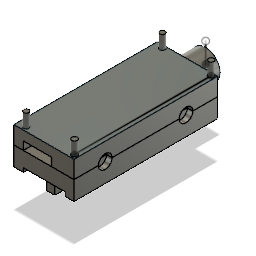
Atari 7800 mod Stand v7 (Autodesk Fusion 360 design; units mm, degrees)
Autodesk Fusion 360 part; units mm, degrees
sketch "Sketch1" plane through (0, 0, 0) normal (0, 1, 0) x (1, 0, 0)
  circle A0 centre (10, -10) radius 1
  circle A1 centre (26.65, -10) radius 1
  circle A2 centre (26.65, -58.45) radius 1
  circle A3 centre (10, -58.45) radius 1
  dimension "d1" = 2
  dimension "d3" = 16.65
  dimension "d4" = 2
  dimension "d5" = 48.45
  dimension "d6" = 2
  dimension "d7" = 2
  measures "d1" diameter of A0
  measures "d3" distance of A0.centre A1.centre
  measures "d4" diameter of A1
  measures "d5" distance of A1.centre A2.centre
  measures "d6" diameter of A2
  measures "d7" diameter of A3
extrude "Extrude1" add sketch "Sketch1" along normal blind 5 makes body 1 at (27.6488, 3.3333, 10.0498) makes body 2 at (9.0603, 3.3333, 58.792) makes body 3 at (10.9988, 3.3333, 10.0498) makes body 4 at (27.5897, 3.3333, 58.792)
sketch "Sketch3" plane through (0, 0, 0) normal (0, 1, 0) x (1, 0, 0)
  line L0 (9, -9) -> (28, -9)
  line L1 (28, -9) -> (28, -60)
  line L2 (28, -60) -> (9, -60)
  line L3 (9, -60) -> (9, -9)
  constraint horizontal L0
  constraint vertical L1
  constraint horizontal L2
  constraint vertical L3
extrude "Extrude2" add sketch "Sketch3" against normal blind 1 bodies 1 2 3 4
sketch "Sketch6" plane through (0, 0, 9) normal (0, 0, -1) x (-1, 0, 0)
  line L0 (-9, 0) -> (-10, 0)
  line L1 (-10, 0) -> (-26.65, 0)
  line L2 (-26.65, 0) -> (-28, 0)
  line L3 (-28, 0) -> (-28, -1)
  line L4 (-28, -1) -> (-9, -1)
  line L5 (-9, -1) -> (-9, 0)
  line L6 (-25.65, 0) -> (-14.65, 0)
  line L7 (-14.65, 0) -> (-14.65, -2)
  circle A0 centre (-14.65, -7.3) radius 5.3
  point P0 (-25.65, 0)
  dimension "d12" = 11
  dimension "d13" = 2
  dimension "d14" = 10.6
  constraint coincident P0 L6.start
  constraint coincident L7.end A0
  measures "d12" distance of P0 L6.end
  measures "d13" distance of L6.end L7.end
  measures "d14" diameter of A0
extrude "Extrude3" add sketch "Sketch6" against normal blind 24.4 separate body contours A0 makes body 5
sketch "Sketch7" plane through (0, 0, 33.4) normal (0, 0, 1) x (1, 0, 0)
  circle A0 centre (14.65, -7.3) radius 5.3
  circle A1 centre (14.65, -7.3) radius 4.625
  circle A2 centre (14.65, -7.3) radius 3.85
  line L0 (14.65, -7.3) -> (19.275, -7.3)
  line L1 (14.65, -7.3) -> (10.025, -7.3)
  line L2 (10.025, -7.3) -> (14.65, -7.3)
  line L3 (14.65, -7.3) -> (14.65, -2.675)
  line L4 (14.65, -7.3) -> (14.65, -11.925)
  line L5 (14.65, -3.45) -> (12.0872, -3.45)
  line L6 (12.0872, -3.45) -> (14.65, -3.45)
  line L7 (17.2128, -3.45) -> (14.65, -3.45)
  line L8 (14.65, -11.15) -> (17.2128, -11.15)
  line L9 (14.65, -11.15) -> (12.0872, -11.15)
  constraint concentric A0 A1
  constraint concentric A1 A2
  constraint coincident A0.centre A1.centre
  constraint coincident A1 L0.end
  constraint coincident A1 L1.end
  constraint parallel L0 L1
  constraint coincident A1 L3.end
  constraint perpendicular L0 L3
  constraint coincident A1 L4.end
  constraint perpendicular L2 L4
  constraint coincident A2 L5.start
  constraint coincident L3 L5.start
  constraint coincident A1 L5.end
  constraint tangent A2 L5
  constraint coincident A1 L7.start
  constraint tangent A2 L7
  constraint coincident A2 L8.start
  constraint coincident L4 L8.start
  constraint coincident A1 L8.end
  constraint tangent A2 L8
  constraint coincident A1 L9.end
  constraint tangent A2 L9
extrude "Extrude4" add sketch "Sketch7" along normal blind 13 contours A1 A2 L0 L7 | A1 A2 L0 L8 | A2 L0 L3 | A2 L0 L4 | A2 L1 L2 L3 | A1 A2 L1 L2 L5 L6 | A1 A2 L1 L2 L9 | A2 L1 L2 L4 bodies 5
sketch "Sketch8" plane through (0, -11.15, 0) normal (0, -1, 0) x (1, 0, 0)
  line L0 (12.0872, 33.4) -> (17.2128, 33.4)
  line L1 (17.2128, 33.4) -> (17.2128, 46.4)
  line L2 (17.2128, 46.4) -> (12.0872, 46.4)
  line L3 (12.0872, 46.4) -> (12.0872, 33.4)
  line L4 (14.65, 46.4) -> (14.65, 44.4)
  line L5 (14.65, 33.4) -> (14.65, 37.4)
  line L6 (14.65, 37.4) -> (19.65, 37.4)
  line L7 (19.65, 37.4) -> (19.65, 38.7)
  line L8 (19.65, 38.7) -> (14.65, 38.7)
  line L9 (14.65, 38.7) -> (14.65, 37.4)
  line L10 (14.65, 44.4) -> (19.65, 44.4)
  line L11 (19.65, 44.4) -> (19.65, 43.1)
  line L12 (19.65, 43.1) -> (14.65, 43.1)
  line L13 (14.65, 43.1) -> (14.65, 44.4)
  line L14 (14.65, 41.5) -> (19.65, 41.5)
  line L15 (19.65, 41.5) -> (19.65, 40.2)
  line L16 (19.65, 40.2) -> (14.65, 40.2)
  line L17 (14.65, 40.2) -> (14.65, 41.5)
  line L18 (14.65, 44.4) -> (9.65, 44.4)
  line L19 (9.65, 44.4) -> (9.65, 43.1)
  line L20 (9.65, 43.1) -> (14.65, 43.1)
  line L21 (14.65, 43.1) -> (14.65, 44.4)
  line L22 (14.65, 41.5) -> (9.65, 41.5)
  line L23 (9.65, 41.5) -> (9.65, 40.2)
  line L24 (9.65, 40.2) -> (14.65, 40.2)
  line L25 (14.65, 40.2) -> (14.65, 41.5)
  line L26 (14.65, 38.7) -> (9.65, 38.7)
  line L27 (9.65, 38.7) -> (9.65, 37.4)
  line L28 (9.65, 37.4) -> (14.65, 37.4)
  line L29 (14.65, 37.4) -> (14.65, 38.7)
  dimension "d21" = 2
  dimension "d26" = 4
  dimension "d27" = 5
  dimension "d28" = 1.3
  dimension "d29" = 5
  dimension "d30" = 1.3
  dimension "d31" = 1.6
  dimension "d32" = 5
  dimension "d33" = 1.3
  dimension "d34" = 5
  dimension "d35" = 5
  dimension "d36" = 1.3
  dimension "d37" = 1.3
  dimension "d38" = 5
  constraint midpoint L2 L4.start
  constraint midpoint L0 L5.start
  constraint horizontal L6
  constraint vertical L7
  constraint horizontal L8
  constraint vertical L9
  constraint horizontal L10
  constraint vertical L11
  constraint horizontal L12
  constraint vertical L13
  constraint horizontal L14
  constraint vertical L15
  constraint horizontal L16
  constraint vertical L17
  constraint horizontal L18
  constraint vertical L19
  constraint horizontal L20
  constraint vertical L21
  constraint horizontal L22
  constraint vertical L23
  constraint horizontal L24
  constraint vertical L25
  constraint horizontal L26
  constraint vertical L27
  constraint horizontal L28
  constraint vertical L29
  measures "d21" distance of L4.start L4.end
  measures "d26" distance of L5.start L5.end
  measures "d27" distance of L5.end L6.end
  measures "d28" distance of L5.end L8.end
  measures "d29" distance of L4.end L10.end
  measures "d30" distance of L4.end L12.end
  measures "d31" distance of L12.end L14.start
  measures "d32" distance of L14.start L14.end
  measures "d33" distance of L14.start L16.end
  measures "d34" distance of L4.end L18.end
  measures "d35" distance of L14.start L22.end
  measures "d36" distance of L14.start L16.end
  measures "d37" distance of L8.end L5.end
  measures "d38" distance of L8.end L26.end
extrude "Extrude5" cut sketch "Sketch8" against normal blind 3 contours L3 L26 L27 L28 | L3 L9 L26 L28 L29 | L1 L6 L8 L9 L29 | L1 L6 L7 L8 | L3 L22 L23 L24 | L3 L17 L22 L24 L25 | L1 L14 L16 L17 L25 | L1 L14 L15 L16 | L3 L18 L19 L20 | L3 L13 L18 L20 L21 | L1 L10 L12 L13 L21 | L1 L10 L11 L12 bodies 5
sketch "Sketch9" plane through (0, -3.45, 0) normal (0, 1, 0) x (-1, 0, 0)
  line L0 (-17.2128, 33.4) -> (-12.0872, 33.4)
  line L1 (-12.0872, 33.4) -> (-12.0872, 46.4)
  line L2 (-12.0872, 46.4) -> (-17.2128, 46.4)
  line L3 (-17.2128, 46.4) -> (-17.2128, 33.4)
  line L4 (-19.1962, 44.4) -> (-10.1038, 44.4)
  line L5 (-10.1038, 44.4) -> (-10.1038, 43.1)
  line L6 (-10.1038, 43.1) -> (-19.1962, 43.1)
  line L7 (-19.1962, 43.1) -> (-19.1962, 44.4)
  line L8 (-10.1038, 41.5) -> (-19.1962, 41.5)
  line L9 (-19.1962, 41.5) -> (-19.1962, 40.2)
  line L10 (-19.1962, 40.2) -> (-10.1038, 40.2)
  line L11 (-10.1038, 40.2) -> (-10.1038, 41.5)
  line L12 (-19.1962, 38.7) -> (-10.1038, 38.7)
  line L13 (-10.1038, 38.7) -> (-10.1038, 37.4)
  line L14 (-10.1038, 37.4) -> (-19.1962, 37.4)
  line L15 (-19.1962, 37.4) -> (-19.1962, 38.7)
  point P0 (-19.1962, 44.4)
  point P1 (-10.1038, 43.1)
  point P2 (-10.1038, 41.5)
  point P3 (-19.1962, 40.2)
  point P4 (-19.1962, 38.7)
  point P5 (-10.1038, 37.4)
  constraint horizontal L4
  constraint vertical L5
  constraint horizontal L6
  constraint vertical L7
  constraint coincident P1 L5.end
  constraint coincident P0 L4.start
  constraint horizontal L8
  constraint vertical L9
  constraint horizontal L10
  constraint vertical L11
  constraint coincident P3 L9.end
  constraint coincident P2 L8.start
  constraint horizontal L12
  constraint vertical L13
  constraint horizontal L14
  constraint vertical L15
  constraint coincident P5 L13.end
  constraint coincident P4 L12.start
extrude "Extrude6" cut sketch "Sketch9" against normal blind 3 contours L3 L12 L14 L15 | L1 L3 L12 L14 | L1 L12 L13 L14 | L3 L8 L9 L10 | L1 L3 L8 L10 | L1 L8 L10 L11 | L3 L4 L6 L7 | L1 L3 L4 L6 | L1 L4 L5 L6 bodies 5
move_body "Move2" bodies 5 to x (1, 0, 0) y (0, 1, 0) z (0, 0, 1) at (0, 0, -9)
sketch "Sketch10" plane through (0, 5, 0) normal (0, 1, 0) x (-1, 0, 0)
  circle A0 centre (-26.65, 10) radius 1
sketch "Sketch11" plane through (0, 0, 0) normal (0, 0, 1) x (1, 0, 0)
  line L0 (5, 5) -> (5, -23.5)
  line L1 (5, -23.5) -> (35, -23.5)
  line L2 (35, -23.5) -> (35, -25)
  line L3 (35, -25) -> (5, -25)
  line L4 (5, -25) -> (5, -23.5)
  dimension "d43" = 28.5
  dimension "d44" = 30
  constraint horizontal L1
  constraint vertical L2
  constraint horizontal L3
  constraint vertical L4
  measures "d43" distance of L0.start L0.end
  measures "d44" distance of L0.end L1.end
extrude "Extrude7" add sketch "Sketch11" along normal blind 66 separate body makes body 6
extrude "Extrude8" add 1 faces at (15.3333, -1, 26) along direction (0, -1, 0) blind 1 on bodies 1 bodies 1
sketch "Sketch12" plane through (0, 0, 60) normal (0, 0, 1) x (1, 0, 0)
  line L0 (28, 0) -> (9, 0)
  line L1 (9, 0) -> (9, -2)
  line L2 (9, -2) -> (28, -2)
  line L3 (28, -2) -> (28, 0)
  line L4 (9, -2) -> (17.2128, -2)
  line L5 (17.2128, -2) -> (17.2128, -3.45)
  line L6 (17.2128, -3.45) -> (9, -3.45)
  line L7 (9, -3.45) -> (9, -2)
  line L8 (17.2128, -3.45) -> (28, -3.45)
  line L9 (28, -3.45) -> (28, -2)
  line L10 (28, -2) -> (17.2128, -2)
  line L11 (17.2128, -2) -> (17.2128, -3.45)
  point P0 (17.2128, -3.45)
  point P1 (17.2128, -3.45)
  constraint horizontal L4
  constraint vertical L5
  constraint horizontal L6
  constraint vertical L7
  constraint coincident P1 P0
  constraint coincident L1.end L2.start
  constraint horizontal L8
  constraint vertical L9
  constraint horizontal L10
  constraint vertical L11
  constraint coincident L2.end L3.start
extrude "Extrude9" add sketch "Sketch12" against normal blind 35 contours L2 L5 L8 L9 L10 L11 | L2 L4 L5 L6 L7 L11 bodies 1
sketch "Sketch13" plane through (0, -3.45, 0) normal (0, -1, 0) x (1, 0, 0)
  line L0 (28, 60) -> (9, 60)
  line L1 (9, 60) -> (9, 25)
  line L2 (9, 25) -> (28, 25)
  line L3 (28, 25) -> (28, 60)
  line L4 (9, 25) -> (10, 25)
  line L5 (10, 25) -> (10, 60)
  line L6 (10, 60) -> (9, 60)
  line L7 (9, 60) -> (9, 25)
  line L8 (28, 25) -> (19.3, 25)
  line L9 (19.3, 25) -> (19.3, 35.4)
  line L10 (19.3, 35.4) -> (28, 35.4)
  line L11 (28, 35.4) -> (28, 25)
  line L12 (19.3, 35.4) -> (28, 35.4)
  line L13 (28, 35.4) -> (28, 60)
  line L14 (28, 60) -> (19.3, 60)
  line L15 (19.3, 60) -> (19.3, 35.4)
  constraint horizontal L4
  constraint vertical L5
  constraint horizontal L6
  constraint vertical L7
  constraint coincident L0 L5.end
  constraint coincident L1.end L2.start
  constraint horizontal L8
  constraint vertical L9
  constraint horizontal L10
  constraint vertical L11
  constraint coincident L2.end L3.start
  constraint horizontal L12
  constraint vertical L13
  constraint horizontal L14
  constraint vertical L15
  constraint coincident L0.start L3.end
extrude "Extrude10" add sketch "Sketch13" along normal blind 4 contours L0 L3 L10 L12 L13 L14 L15 | L2 L3 L8 L9 L10 L11 L12 | L0 L1 L2 L4 L5 L6 L7 bodies 1
sketch "Sketch14" plane through (0, 0, 9) normal (0, 0, -1) x (-1, 0, 0)
  line L0 (-9, 0) -> (-10, 0)
  line L1 (-10, 0) -> (-26.65, 0)
  line L2 (-26.65, 0) -> (-28, 0)
  line L3 (-28, 0) -> (-28, -2)
  line L4 (-28, -2) -> (-9, -2)
  line L5 (-9, -2) -> (-9, 0)
  line L6 (-9, -2) -> (-28, -2)
  line L7 (-28, -2) -> (-28, -7.45)
  line L8 (-28, -7.45) -> (-9, -7.45)
  line L9 (-9, -7.45) -> (-9, -2)
  circle A0 centre (-14.65, -7.2999) radius 5.3001
  circle A1 centre (-14.65, -7.3) radius 5.3
  point P0 (-28, -7.45)
  constraint horizontal L6
  constraint vertical L7
  constraint horizontal L8
  constraint vertical L9
  constraint coincident P0 L7.end
  constraint coincident L4.end L5.start
  constraint tangent A0 A1
extrude "Extrude11" add sketch "Sketch14" against normal blind 16 contours L4 L6 L8 L9 A0 A1 | L4 L6 L7 L8 A0 A1 bodies 1
sketch "Sketch15" plane through (0, -3.45, 0) normal (0, -1, 0) x (1, 0, 0)
  line L0 (10, 60) -> (10, 25)
  line L1 (10, 25) -> (11.0072, 25)
  line L2 (11.0072, 25) -> (18.2928, 25)
  line L3 (18.2928, 25) -> (19.3, 25)
  line L4 (19.3, 25) -> (19.3, 60)
  line L5 (19.3, 60) -> (10, 60)
  line L6 (10.1038, 35.4) -> (19.1962, 35.4)
  line L7 (19.1962, 35.4) -> (19.1962, 34.1)
  line L8 (19.1962, 34.1) -> (10.1038, 34.1)
  line L9 (10.1038, 34.1) -> (10.1038, 35.4)
  line L10 (19.1962, 32.5) -> (10.1038, 32.5)
  line L11 (10.1038, 32.5) -> (10.1038, 31.2)
  line L12 (10.1038, 31.2) -> (19.1962, 31.2)
  line L13 (19.1962, 31.2) -> (19.1962, 32.5)
  line L14 (10.1038, 29.7) -> (19.1962, 29.7)
  line L15 (19.1962, 29.7) -> (19.1962, 28.4)
  line L16 (19.1962, 28.4) -> (10.1038, 28.4)
  line L17 (10.1038, 28.4) -> (10.1038, 29.7)
  point P0 (10.1038, 35.4)
  point P1 (19.1962, 34.1)
  point P2 (19.1962, 32.5)
  point P3 (10.1038, 31.2)
  point P4 (10.1038, 29.7)
  point P5 (19.1962, 28.4)
  constraint horizontal L6
  constraint vertical L7
  constraint horizontal L8
  constraint vertical L9
  constraint coincident P1 L7.end
  constraint coincident P0 L6.start
  constraint horizontal L10
  constraint vertical L11
  constraint horizontal L12
  constraint vertical L13
  constraint coincident P3 L11.end
  constraint coincident P2 L10.start
  constraint horizontal L14
  constraint vertical L15
  constraint horizontal L16
  constraint vertical L17
  constraint coincident P5 L15.end
  constraint coincident P4 L14.start
extrude "Extrude12" add sketch "Sketch15" along normal blind 3 contours L6 L7 L8 L9 | L10 L11 L12 L13 | L14 L15 L16 L17 bodies 1
extrude "Extrude13" cut 4 faces at (9.4507, -7.45, 48.3333) (9.1174, -7.45, 14.3333) (22.416, -7.45, 48.3333) (25.316, -7.45, 14.3333) along direction (0, 1, 0) blind 1 on bodies 1 bodies 1
sketch "Sketch16" plane through (0, 0, 9) normal (0, 0, -1) x (-1, 0, 0)
  line L0 (-9.352, -6.45) -> (-9, -6.45)
  line L1 (-9, -6.45) -> (-9, 0)
  line L2 (-9, 0) -> (-10, 0)
  line L3 (-10, 0) -> (-26.65, 0)
  line L4 (-26.65, 0) -> (-28, 0)
  line L5 (-28, 0) -> (-28, -6.45)
  line L6 (-28, -6.45) -> (-19.948, -6.45)
  line L7 (-19.948, -6.45) -> (-19.948, -7.1498)
  arc A0 (-14.7005, -2) -> (-19.948, -7.1498) centre (-14.65, -7.2999) ccw
  line L8 (-14.7005, -2) -> (-14.5995, -2)
  arc A1 (-9.352, -7.1498) -> (-14.5995, -2) centre (-14.65, -7.2999) ccw
  line L9 (-9.352, -7.1498) -> (-9.352, -6.45)
  line L10 (-9, -6.45) -> (-21.6476, -6.45)
  line L11 (-21.6476, -6.45) -> (-21.6476, -7.1824)
  line L12 (-21.6476, -7.1824) -> (-9, -7.1824)
  line L13 (-9, -7.1824) -> (-9, -6.45)
  constraint horizontal L10
  constraint vertical L11
  constraint horizontal L12
  constraint vertical L13
  constraint coincident L0.end L1.start
extrude "Extrude14" cut 1 faces at (9.3521, -6.9152, 19.6667) along direction (1, 0, 0) blind 1 on bodies 1 bodies 1
extrude "Extrude15" cut 1 faces at (19.9479, -6.9151, 19.6667) along direction (-1, 0, 0) blind 1 on bodies 1 bodies 1
sketch "Sketch17" plane through (0, -6.45, 0) normal (0, -1, 0) x (1, 0, 0)
  line L0 (28, 9) -> (28, 60)
  line L1 (28, 60) -> (19.3, 60)
  line L2 (19.3, 60) -> (19.3, 25)
  line L3 (19.3, 25) -> (19.8815, 25)
  line L4 (19.8815, 25) -> (19.8815, 9)
  line L5 (19.8815, 9) -> (28, 9)
  line L6 (28, 9) -> (19.3, 9)
  line L7 (19.3, 9) -> (19.3, 60)
  line L8 (19.3, 60) -> (28, 60)
  line L9 (28, 60) -> (28, 9)
  line L10 (9, 9) -> (10, 9)
  line L11 (10, 9) -> (10, 60)
  line L12 (10, 60) -> (9, 60)
  line L13 (9, 60) -> (9, 9)
  point P0 (9, 9)
  point P1 (10, 60)
  constraint horizontal L6
  constraint vertical L7
  constraint horizontal L8
  constraint vertical L9
  constraint coincident L1.end L2.start
  constraint coincident L0.start L5.end
  constraint horizontal L10
  constraint vertical L11
  constraint horizontal L12
  constraint vertical L13
  constraint coincident P1 L11.end
  constraint coincident P0 L10.start
extrude "Extrude16" add sketch "Sketch17" along normal blind 2 separate body contours L0 L1 L2 L3 L4 L5 L6 L7 L8 L9 | L10 L11 L12 L13 makes body 7 at (25.2938, -6.45, 31.3333) makes body 8 at (9, -7.1167, 43)
sketch "Sketch18" plane through (0, -8.45, 0) normal (0, -1, 0) x (1, 0, 0)
  line L0 (19.3, 25) -> (19.8815, 25)
  line L1 (19.8815, 25) -> (19.8815, 9)
  line L2 (19.8815, 9) -> (28, 9)
  line L3 (28, 9) -> (28, 60)
  line L4 (28, 60) -> (19.3, 60)
  line L5 (19.3, 60) -> (19.3, 25)
  line L6 (19.1962, 35.4) -> (19.1962, 34.1)
  line L7 (19.1962, 34.75) -> (28, 34.7618)
  line L8 (28, 34.7618) -> (28, 35.2618)
  line L9 (28, 35.2618) -> (9, 35.2618)
  line L10 (9, 35.2618) -> (9, 34.2618)
  line L11 (9, 34.2618) -> (28, 34.2618)
  line L12 (28, 34.2618) -> (28, 35.2618)
  line L13 (19.1962, 32.5) -> (10.1038, 32.5)
  line L14 (10.1038, 32.5) -> (10.1038, 31.2)
  line L15 (10.1038, 31.2) -> (19.1962, 31.2)
  line L16 (10.1038, 29.7) -> (19.1962, 29.7)
  line L17 (19.1962, 28.4) -> (10.1038, 28.4)
  line L18 (10.1038, 28.4) -> (10.1038, 29.7)
  line L19 (19.1962, 31.85) -> (28, 31.8539)
  line L20 (19.1962, 29.05) -> (28, 29)
  line L21 (28, 29) -> (28, 29.5)
  line L22 (28, 31.8539) -> (28, 32.3539)
  line L23 (28, 29.5) -> (9, 29.5)
  line L24 (9, 29.5) -> (9, 28.5)
  line L25 (9, 28.5) -> (28, 28.5)
  line L26 (28, 28.5) -> (28, 29.5)
  line L27 (28, 32.3539) -> (9, 32.3539)
  line L28 (9, 32.3539) -> (9, 31.3539)
  line L29 (9, 31.3539) -> (28, 31.3539)
  line L30 (28, 31.3539) -> (28, 32.3539)
  line L31 (9, 60) -> (10, 60)
  line L32 (10, 60) -> (10, 9)
  line L33 (10, 9) -> (9, 9)
  line L34 (9, 9) -> (9, 60)
  point P0 (19.1962, 32.5)
  point P1 (10.1038, 31.2)
  point P2 (10.1038, 29.7)
  point P3 (19.1962, 28.4)
  point P4 (9, 60)
  point P5 (10, 9)
  dimension "d65" = 0.5
  dimension "d66" = 1
  dimension "d67" = 0.5
  dimension "d68" = 0.5
  dimension "d69" = 1
  dimension "d70" = 1
  constraint midpoint L6 L7.start
  constraint coincident L3 L7.end
  constraint horizontal L9
  constraint vertical L10
  constraint horizontal L11
  constraint vertical L12
  constraint horizontal L13
  constraint vertical L14
  constraint horizontal L15
  constraint coincident P1 L14.end
  constraint coincident P0 L13.start
  constraint horizontal L16
  constraint horizontal L17
  constraint vertical L18
  constraint coincident P3 L17.start
  constraint coincident P2 L16.start
  constraint coincident L3 L19.end
  constraint coincident L3 L20.end
  constraint horizontal L23
  constraint vertical L24
  constraint horizontal L25
  constraint vertical L26
  constraint horizontal L27
  constraint vertical L28
  constraint horizontal L29
  constraint vertical L30
  constraint horizontal L31
  constraint vertical L32
  constraint horizontal L33
  constraint vertical L34
  constraint coincident P5 L32.end
  constraint coincident P4 L31.start
  measures "d65" distance of L7.end L8.end
  measures "d66" distance of L8.end L11.end
  measures "d67" distance of L20.end L21.end
  measures "d68" distance of L19.end L22.end
  measures "d69" distance of L21.end L25.end
  measures "d70" distance of L22.end L29.end
extrude "Extrude17" add sketch "Sketch18" along normal blind 3 contours L0 L1 L2 L3 L5 L25 | L5 L18 L23 L25 | L3 L5 L20 L25 L26 | L3 L5 L20 L21 L23 L26 | L3 L5 L23 L29 | L25 L32 L33 L34 | L23 L24 L25 L32 L34 | L5 L14 L27 L29 | L3 L5 L19 L29 L30 | L23 L29 L32 L34 | L3 L5 L19 L22 L27 L30 | L27 L28 L29 L32 L34 | L3 L5 L11 L27 | L11 L27 L32 L34 | L3 L5 L7 L11 L12 | L6 L9 L11 L32 | L9 L10 L11 L32 L34 | L3 L5 L7 L8 L9 L12 | L9 L31 L32 L34 | L3 L4 L5 L9 bodies 8 makes body 9 at (25.1, -8.45, 33.7846)
extrude "Extrude18" add 1 faces at (10.1038, -9.45, 32.0206) along direction (-1, 0, 0) blind 1 on bodies 9 bodies 9 8
extrude "Extrude19" add 1 faces at (10.1038, -9.45, 28.8333) along direction (-1, 0, 0) blind 0.3 on bodies 9 bodies 9
extrude "Extrude20" add 1 faces at (19.1962, -9.45, 34.9285) along direction (1, 0, 0) blind 0.3 on bodies 9 bodies 9
extrude "Extrude21" add 1 faces at (25.2938, -8.45, 31.3333) along direction (0, -1, 0) blind 1 on bodies 7 bodies 7 9
sketch "Sketch19" plane through (19.3, 0, 0) normal (-1, 0, 0) x (0, 0, 1)
  line L0 (60, -11.45) -> (60, -6.45)
  line L1 (60, -6.45) -> (25, -6.45)
  line L2 (25, -6.45) -> (25, -11.45)
  line L3 (25, -11.45) -> (28.5, -11.45)
  line L4 (28.5, -11.45) -> (28.5, -8.45)
  line L5 (28.5, -8.45) -> (29.5, -8.45)
  line L6 (29.5, -8.45) -> (29.5, -11.45)
  line L7 (29.5, -11.45) -> (31.3539, -11.45)
  line L8 (31.3539, -11.45) -> (31.3539, -8.45)
  line L9 (31.3539, -8.45) -> (32.3539, -8.45)
  line L10 (32.3539, -8.45) -> (32.3539, -11.45)
  line L11 (32.3539, -11.45) -> (34.2618, -11.45)
  line L12 (34.2618, -11.45) -> (34.2618, -8.45)
  line L13 (34.2618, -8.45) -> (35.2618, -8.45)
  line L14 (35.2618, -8.45) -> (35.2618, -11.45)
  line L15 (35.2618, -11.45) -> (60, -11.45)
  line L16 (60, -11.45) -> (58, -11.45)
  line L17 (58, -11.45) -> (58, -6.45)
  line L18 (58, -6.45) -> (60, -6.45)
  line L19 (60, -6.45) -> (60, -11.45)
  dimension "d81" = 2
  constraint horizontal L16
  constraint vertical L17
  constraint horizontal L18
  constraint vertical L19
  constraint coincident L0.start L15.end
  measures "d81" distance of L0.start L16.end
extrude "Extrude22" add sketch "Sketch19" along normal blind 10 contours L0 L1 L15 L16 L17 L18 L19 bodies 7
sketch "Sketch20" plane through (28, 0, 0) normal (1, 0, 0) x (0, 0, -1)
  line L0 (-60, -6.45) -> (-9, -6.45)
  line L1 (-9, -6.45) -> (-9, 0)
  line L2 (-9, 0) -> (-60, 0)
  line L3 (-60, 0) -> (-60, -6.45)
  circle A0 centre (-50.0734, -6.45) radius 2.5
  circle A1 centre (-20.5371, -6.45) radius 2.5
  dimension "d84" = 5
  dimension "d85" = 5
  constraint coincident L0 A0.centre
  constraint coincident L0 A1.centre
  measures "d84" diameter of A0
  measures "d85" diameter of A1
extrude "Extrude23" cut sketch "Sketch20" against normal blind 2 contours L0 A1 | L0 A1 | L0 A0 | L0 A0 bodies 1 7
sketch "Sketch21" plane through (9, 0, 0) normal (-1, 0, 0) x (0, 0, 1)
  line L0 (60, -6.45) -> (9, -6.45)
  line L1 (9, -6.45) -> (9, -11.45)
  line L2 (9, -11.45) -> (60, -11.45)
  line L3 (60, -11.45) -> (60, -6.45)
  circle A0 centre (52.5734, -6.45) radius 2.5
  circle A1 centre (18.0371, -6.45) radius 2.5
  point P0 (52.5734, -6.45)
  point P1 (18.0371, -6.45)
  dimension "d88" = 5
  dimension "d89" = 5
  constraint coincident P0 A0.centre
  constraint coincident P1 A1.centre
  measures "d88" diameter of A0
  measures "d89" diameter of A1
extrude "Extrude24" cut sketch "Sketch21" against normal blind 0.7 contours L0 A0 | L0 A0 bodies 1 7
extrude "Extrude25" add 1 faces at (25.2938, -11.45, 31.3333) along direction (0, -1, 0) blind 2 on bodies 7 bodies 7
sketch "Sketch22" plane through (0, -13.45, 0) normal (0, -1, 0) x (1, 0, 0)
  line L0 (28, 60) -> (9, 60)
  line L1 (9, 60) -> (9, 9)
  line L2 (9, 9) -> (10, 9)
  line L3 (10, 9) -> (10, 28.5)
  line L4 (10, 28.5) -> (19.3, 28.5)
  line L5 (19.3, 28.5) -> (19.3, 25)
  line L6 (19.3, 25) -> (19.8815, 25)
  line L7 (19.8815, 25) -> (19.8815, 9)
  line L8 (19.8815, 9) -> (28, 9)
  line L9 (28, 9) -> (28, 60)
  line L10 (10, 29.5) -> (10, 31.3539)
  line L11 (10, 31.3539) -> (19.3, 31.3539)
  line L12 (19.3, 31.3539) -> (19.3, 29.5)
  line L13 (19.3, 29.5) -> (10, 29.5)
  line L14 (10, 34.2618) -> (19.3, 34.2618)
  line L15 (19.3, 34.2618) -> (19.3, 32.3539)
  line L16 (19.3, 32.3539) -> (10, 32.3539)
  line L17 (10, 32.3539) -> (10, 34.2618)
  line L18 (10, 58) -> (19.3, 58)
  line L19 (19.3, 58) -> (19.3, 35.2618)
  line L20 (19.3, 35.2618) -> (10, 35.2618)
  line L21 (10, 35.2618) -> (10, 58)
  line L22 (10, 60) -> (23.7, 60)
  line L23 (23.7, 60) -> (23.7, 34.3)
  line L24 (23.7, 34.3) -> (10, 34.3)
  line L25 (10, 34.3) -> (10, 60)
  point P0 (10, 60)
  dimension "d94" = 13.7
  dimension "d95" = 25.7
  constraint horizontal L22
  constraint vertical L23
  constraint horizontal L24
  constraint vertical L25
  constraint coincident P0 L22.start
  measures "d94" distance of P0 L22.end
  measures "d95" distance of P0 L24.end
extrude "Extrude26" cut sketch "Sketch22" against normal blind 1.5 contours L0 L18 L19 L20 L22 L23 L24 L25 | L18 L19 L20 L21 L25 bodies 7
sketch "Sketch23" plane through (0, -13.45, 0) normal (0, -1, 0) x (1, 0, 0)
  line L0 (10, 34.3) -> (10, 60)
  line L1 (10, 60) -> (9, 60)
  line L2 (9, 60) -> (9, 9)
  line L3 (9, 9) -> (10, 9)
  line L4 (10, 9) -> (10, 28.5)
  line L5 (10, 28.5) -> (19.3, 28.5)
  line L6 (19.3, 28.5) -> (19.3, 25)
  line L7 (19.3, 25) -> (19.8815, 25)
  line L8 (19.8815, 25) -> (19.8815, 9)
  line L9 (19.8815, 9) -> (28, 9)
  line L10 (28, 9) -> (28, 60)
  line L11 (28, 60) -> (23.7, 60)
  line L12 (23.7, 60) -> (23.7, 34.3)
  line L13 (23.7, 34.3) -> (10, 34.3)
  line L14 (10, 29.5) -> (10, 31.3539)
  line L15 (10, 31.3539) -> (19.3, 31.3539)
  line L16 (19.3, 31.3539) -> (19.3, 29.5)
  line L17 (19.3, 29.5) -> (10, 29.5)
  line L18 (10, 34.2618) -> (19.3, 34.2618)
  line L19 (19.3, 34.2618) -> (19.3, 32.3539)
  line L20 (19.3, 32.3539) -> (10, 32.3539)
  line L21 (10, 32.3539) -> (10, 34.2618)
  line L22 (19.3, 34.2618) -> (10, 34.2618)
  line L23 (10, 34.2618) -> (10, 28.5)
  line L24 (10, 28.5) -> (19.3, 28.5)
  line L25 (19.3, 28.5) -> (19.3, 34.2618)
  line L26 (19.3, 34.2618) -> (10, 34.2618)
  line L27 (10, 34.2618) -> (10, 34.3)
  line L28 (10, 34.3) -> (19.3, 34.3)
  line L29 (19.3, 34.3) -> (19.3, 34.2618)
  constraint horizontal L22
  constraint vertical L23
  constraint horizontal L24
  constraint vertical L25
  constraint coincident L4.end L5.start
  constraint coincident L18.end L19.start
  constraint horizontal L26
  constraint vertical L27
  constraint horizontal L28
  constraint vertical L29
  constraint coincident L0.start L13.end
extrude "Extrude27" cut sketch "Sketch23" against normal blind 1.5 contours L13 L18 L22 L26 L27 L28 L29 | L18 L19 L20 L21 L22 L23 L25 L26 | L15 L20 L23 L25 | L14 L15 L16 L17 L23 L25 | L5 L17 L23 L24 L25 bodies 7
sketch "Sketch24" plane through (0, 0, 9) normal (0, 0, -1) x (-1, 0, 0)
  line L0 (-19.8815, -13.45) -> (-19.8815, -6.45)
  line L1 (-19.8815, -6.45) -> (-28, -6.45)
  line L2 (-28, -6.45) -> (-28, -13.45)
  line L3 (-28, -13.45) -> (-19.8815, -13.45)
  line L4 (-28, -6.45) -> (-9, -6.45)
  line L5 (-9, -6.45) -> (-9, -13.45)
  line L6 (-9, -13.45) -> (-28, -13.45)
  line L7 (-28, -13.45) -> (-28, -6.45)
  circle A0 centre (-14.6632, -7.2997) radius 5.3001
  circle A1 centre (-14.65, -7.3) radius 5.3
  point P0 (-9, -13.45)
  point P1 (-14.5995, -2)
  constraint horizontal L4
  constraint vertical L5
  constraint horizontal L6
  constraint vertical L7
  constraint coincident P0 L5.end
  constraint coincident L1.end L2.start
  constraint coincident A0 P1
extrude "Extrude28" add sketch "Sketch24" against normal blind 16 contours L0 L1 L2 L3 L4 L6 L7 A0 | L0 L4 L5 L6 A0 A1 bodies 7
extrude "Extrude29" cut sketch "Sketch20" against normal blind 2 contours L0 A1 picked at (-20.5624, -7.5266) bodies 7
extrude "Extrude30" add 2 faces at (9, -4.8425, 33.3671) (9, -4.9667, 14.3333) along direction (-1, 0, 0) blind 1 on bodies 1 bodies 1
extrude "Extrude31" add 1 faces at (9, -8.9075, 22.7004) along direction (-1, 0, 0) blind 1 on bodies 7 bodies 7
move_face "MoveFace1" to x (1, 0, 0) y (0, 1, 0) z (0, 0, 1) at (-0.9876, 0, 0.1568) 2 faces at (10, 3.3333, 9) (9.6815, 5, 9.9017) on bodies 1
move_face "MoveFace2" to x (1, 0, 0) y (0, 1, 0) z (0, 0, 1) at (-1, 0, 0) 2 faces at (10.2554, 5, 58.8247) (10.995, 1.6667, 58.3504) on bodies 1
extrude "Extrude32" add 1 faces at (25.1, -3.3, 60) along direction (0, 0, 1) blind 1.5 on bodies 1 bodies 1
move_face "MoveFace3" to x (1, 0, 0) y (0, 1, 0) z (0, 0, 1) at (0, 0, 1.5) 2 faces at (9.2554, 5, 58.8247) (8.0012, 3.3333, 58.4002) on bodies 1
move_face "MoveFace4" to x (1, 0, 0) y (0, 1, 0) z (0, 0, 1) at (0, 0, 1.5) 2 faces at (26.9867, 5, 58.5946) (27.6488, 1.6667, 58.4002) on bodies 1
extrude "Extrude33" add 1 faces at (19.9, -8.2833, 60) along direction (0, 0, 1) blind 1.5 on bodies 7 bodies 7
extrude "Extrude34" cut 1 faces at (23.7, -12.95, 43.3667) along direction (1, 0, 0) blind 1 on bodies 7 bodies 7
sketch "Sketch25" plane through (0, 0, 0) normal (0, 0, -1) x (-1, 0, 0)
  circle A0 centre (-14.65, -7.3) radius 5.3
  circle A1 centre (-14.65, -7.3) radius 5.5
  dimension "d114" = 11
  constraint concentric A0 A1
  measures "d114" diameter of A1
extrude "Extrude35" cut sketch "Sketch25" against normal blind 25 contours A0 | A1 bodies 1 7
extrude "Extrude36" cut 1 faces at (16.1654, -4.45, 28.4) along direction (0, 0, 1) blind 0.15 on bodies 1 bodies 1
extrude "Extrude37" cut 1 faces at (13.1346, -4.45, 31.2) along direction (0, 0, 1) blind 0.15 on bodies 1 bodies 1
extrude "Extrude38" cut 1 faces at (16.1654, -4.45, 34.1) along direction (0, 0, 1) blind 0.15 on bodies 1 bodies 1
extrude "Extrude39" cut 1 faces at (13.1346, -4.45, 29.7) along direction (0, 0, -1) blind 0.15 on bodies 1 bodies 1
extrude "Extrude40" cut 1 faces at (16.1654, -4.45, 32.5) along direction (0, 0, -1) blind 0.15 on bodies 1 bodies 1
extrude "Extrude41" cut 1 faces at (13.1346, -4.45, 35.4) along direction (0, 0, -1) blind 0.15 on bodies 1 bodies 1
extrude "Extrude42" add 3 faces at (10.1038, -4.45, 34.5833) (10.1038, -4.45, 32.0167) (10.1038, -4.45, 28.8833) along direction (-1, 0, 0) blind 1 on bodies 1 bodies 1
extrude "Extrude43" add 3 faces at (19.1962, -4.45, 34.9167) (19.1962, -4.45, 31.6833) (19.1962, -4.45, 29.2167) along direction (1, 0, 0) blind 1 on bodies 1 bodies 1
extrude "Extrude44" cut 4 faces at (10, -4.8855, 27.3667) (10, -4.45, 30.15) (10, -5.45, 33.6167) (10, -4.45, 52.75) along direction (-1, 0, 0) blind 0.5 on bodies 1 bodies 1
extrude "Extrude45" cut 4 faces at (19.3, -4.8855, 27.3667) (19.3, -4.45, 30.15) (19.3, -5.45, 33.6167) (19.3, -4.45, 52.75) along direction (1, 0, 0) blind 0.5 on bodies 1 bodies 1
extrude "Extrude46" cut 1 faces at (19.3, -8.95, 50.4206) along direction (1, 0, 0) blind 0.5 on bodies 7 bodies 7
extrude "Extrude47" cut 1 faces at (10, -8.95, 50.4206) along direction (-1, 0, 0) blind 0.5 on bodies 7 bodies 7
sketch "Sketch26" plane through (9.5, 0, 0) normal (1, 0, 0) x (0, 0, -1)
  line L0 (-28.5, -11.95) -> (-29.5, -11.95)
  line L1 (-29.5, -11.95) -> (-29.5, -8.45)
  line L2 (-29.5, -8.45) -> (-28.5, -8.45)
  line L3 (-28.5, -8.45) -> (-28.5, -11.95)
  line L4 (-31.3539, -11.95) -> (-32.3539, -11.95)
  line L5 (-32.3539, -11.95) -> (-32.3539, -8.45)
  line L6 (-32.3539, -8.45) -> (-31.3539, -8.45)
  line L7 (-31.3539, -8.45) -> (-31.3539, -11.95)
  line L8 (-34.2618, -11.95) -> (-35.2618, -11.95)
  line L9 (-35.2618, -11.95) -> (-35.2618, -8.45)
  line L10 (-35.2618, -8.45) -> (-34.2618, -8.45)
  line L11 (-34.2618, -8.45) -> (-34.2618, -11.95)
  arc A0 (-55.0734, -6.45) -> (-50.0734, -6.45) centre (-52.5734, -6.45) ccw
  line L12 (-55.0734, -6.45) -> (-58, -6.45)
  line L13 (-58, -6.45) -> (-58, -11.95)
  line L14 (-58, -11.95) -> (-61.5, -11.95)
  line L15 (-61.5, -11.95) -> (-61.5, -13.45)
  line L16 (-61.5, -13.45) -> (-25, -13.45)
  line L17 (-25, -13.45) -> (-25, -9.2307)
  line L18 (-25, -9.2307) -> (-25, -6.45)
  line L19 (-25, -6.45) -> (-50.0734, -6.45)
  line L20 (-55.0734, -6.45) -> (-49.0947, -6.45)
  line L21 (-49.0947, -6.45) -> (-49.0947, -9.1965)
  line L22 (-49.0947, -9.1965) -> (-55.0734, -9.1965)
  line L23 (-55.0734, -9.1965) -> (-55.0734, -6.45)
  constraint horizontal L20
  constraint vertical L21
  constraint horizontal L22
  constraint vertical L23
  constraint coincident A0.start L12.start
extrude "Extrude48" add sketch "Sketch26" against normal blind 0.5 contours A0 L20 bodies 7
sketch "Sketch27" plane through (9.5, 0, 0) normal (1, 0, 0) x (0, 0, -1)
  arc A0 (-50.0734, -6.45) -> (-55.0734, -6.45) centre (-52.5734, -6.45) ccw
  line L0 (-50.0734, -6.45) -> (-35.25, -6.45)
  line L1 (-35.25, -6.45) -> (-35.25, -3.45)
  line L2 (-35.25, -3.45) -> (-61.5, -3.45)
  line L3 (-61.5, -3.45) -> (-61.5, -6.45)
  line L4 (-61.5, -6.45) -> (-55.0734, -6.45)
  line L5 (-55.0734, -6.45) -> (-49.9978, -6.45)
  line L6 (-49.9978, -6.45) -> (-49.9978, -3.45)
  line L7 (-49.9978, -3.45) -> (-55.0734, -3.45)
  line L8 (-55.0734, -3.45) -> (-55.0734, -6.45)
  constraint horizontal L5
  constraint vertical L6
  constraint horizontal L7
  constraint vertical L8
  constraint coincident L2 L6.end
  constraint coincident A0.end L4.end
extrude "Extrude49" add sketch "Sketch27" against normal blind 0.5 contours A0 L5 bodies 1
extrude "Extrude50" add 1 faces at (8, -4.1758, 22.7004) along direction (-1, 0, 0) blind 2 on bodies 1 bodies 1
extrude "Extrude51" add 1 faces at (8, -8.9075, 22.7004) along direction (-1, 0, 0) blind 2 on bodies 7 bodies 7
sketch "Sketch28" plane through (6, 0, 0) normal (-1, 0, 0) x (0, 0, 1)
  line L0 (9, -13.45) -> (61.5, -13.45)
  line L1 (61.5, -13.45) -> (61.5, -6.45)
  line L2 (61.5, -6.45) -> (55.0734, -6.45)
  arc A0 (50.0734, -6.45) -> (55.0734, -6.45) centre (52.5734, -6.45) ccw
  line L3 (50.0734, -6.45) -> (9, -6.45)
  line L4 (9, -6.45) -> (9, -13.45)
  line L5 (9, -13.45) -> (22.5, -13.45)
  line L6 (22.5, -13.45) -> (22.5, -26.95)
  line L7 (22.5, -26.95) -> (9, -26.95)
  line L8 (9, -26.95) -> (9, -13.45)
  line L9 (9, -20.2) -> (22.5, -20.2)
  line L10 (22.5, -13.45) -> (36, -13.45)
  line L11 (36, -13.45) -> (36, -26.95)
  line L12 (36, -26.95) -> (22.5, -26.95)
  line L13 (22.5, -26.95) -> (22.5, -13.45)
  line L14 (29.25, -13.45) -> (29.25, -26.95)
  line L15 (36, -13.45) -> (49.5, -13.45)
  line L16 (49.5, -13.45) -> (49.5, -26.95)
  line L17 (49.5, -26.95) -> (36, -26.95)
  line L18 (36, -26.95) -> (36, -13.45)
  line L19 (36, -20.2) -> (49.5, -20.2)
  circle A1 centre (15.75, -20.2) radius 3.1
  circle A2 centre (29.25, -20.2) radius 3.1
  circle A3 centre (42.75, -20.2) radius 3.1
  dimension "d149" = 13.5
  dimension "d150" = 13.5
  dimension "d151" = 13.5
  dimension "d152" = 13.5
  dimension "d153" = 13.5
  dimension "d154" = 13.5
  dimension "d155" = 6.2
  dimension "d156" = 6.2
  dimension "d157" = 6.2
  constraint horizontal L5
  constraint vertical L6
  constraint horizontal L7
  constraint vertical L8
  constraint coincident L0.start L4.end
  constraint midpoint L8 L9.start
  constraint midpoint L6 L9.end
  constraint horizontal L10
  constraint vertical L11
  constraint horizontal L12
  constraint vertical L13
  constraint midpoint L10 L14.start
  constraint midpoint L12 L14.end
  constraint horizontal L15
  constraint vertical L16
  constraint horizontal L17
  constraint vertical L18
  constraint midpoint L11 L19.start
  constraint midpoint L16 L19.end
  constraint midpoint L9 A1.centre
  constraint midpoint L14 A2.centre
  constraint midpoint L19 A3.centre
  measures "d149" distance of L0.start L5.end
  measures "d150" distance of L0.start L7.end
  measures "d151" distance of L5.end L10.end
  measures "d152" distance of L5.end L6.end
  measures "d153" distance of L10.end L15.end
  measures "d154" distance of L10.end L11.end
  measures "d155" diameter of A1
  measures "d156" diameter of A2
  measures "d157" diameter of A3
extrude "Extrude52" add sketch "Sketch28" against normal blind 3 contours L0 L5 L6 L8 L9 L13 A1 | L0 L6 L10 L12 L13 L14 A2 | L6 L7 L8 L9 L13 A1 | L0 L10 L11 L12 L14 L18 A2 | L0 L11 L15 L16 L18 L19 A3 | L11 L16 L17 L18 L19 A3 bodies 7
sketch "Sketch29" plane through (0, -6.45, 0) normal (0, -1, 0) x (1, 0, 0)
  line L0 (9.5, 34.25) -> (19.8, 34.25)
  line L1 (19.8, 34.25) -> (19.8, 32.35)
  line L2 (19.8, 32.35) -> (9.5, 32.35)
  line L3 (9.5, 32.35) -> (9.5, 34.25)
  line L4 (9.5, 31.35) -> (19.8, 31.35)
  line L5 (19.8, 31.35) -> (19.8, 29.55)
  line L6 (19.8, 29.55) -> (9.5, 29.55)
  line L7 (9.5, 29.55) -> (9.5, 31.35)
  line L8 (9.5, 35.25) -> (9.5, 61.5)
  line L9 (9.5, 61.5) -> (6, 61.5)
  line L10 (6, 61.5) -> (6, 55.0734)
  line L11 (6, 55.0734) -> (9, 55.0734)
  line L12 (9, 55.0734) -> (9, 50.0734)
  line L13 (9, 50.0734) -> (6, 50.0734)
  line L14 (6, 50.0734) -> (6, 9)
  line L15 (6, 9) -> (9.2161, 9)
  line L16 (9.2161, 9) -> (9.2161, 25)
  line L17 (9.2161, 25) -> (9.5, 25)
  line L18 (9.5, 25) -> (9.5, 28.55)
  line L19 (9.5, 28.55) -> (19.8, 28.55)
  line L20 (19.8, 28.55) -> (19.8, 25)
  line L21 (19.8, 25) -> (20.0839, 25)
  line L22 (20.0839, 25) -> (20.0839, 9)
  line L23 (20.0839, 9) -> (28, 9)
  line L24 (28, 9) -> (28, 18.0371)
  line L25 (28, 18.0371) -> (26, 18.0371)
  line L26 (26, 18.0371) -> (26, 23.0371)
  line L27 (26, 23.0371) -> (28, 23.0371)
  line L28 (28, 23.0371) -> (28, 47.5734)
  line L29 (28, 47.5734) -> (26, 47.5734)
  line L30 (26, 47.5734) -> (26, 52.5734)
  line L31 (26, 52.5734) -> (28, 52.5734)
  line L32 (28, 52.5734) -> (28, 61.5)
  line L33 (28, 61.5) -> (19.8, 61.5)
  line L34 (19.8, 61.5) -> (19.8, 35.25)
  line L35 (19.8, 35.25) -> (9.5, 35.25)
  line L36 (9.5, 35.25) -> (19.8, 35.25)
  line L37 (19.8, 35.25) -> (19.8, 28.55)
  line L38 (19.8, 28.55) -> (9.5, 28.55)
  line L39 (9.5, 28.55) -> (9.5, 35.25)
  constraint horizontal L36
  constraint vertical L37
  constraint horizontal L38
  constraint vertical L39
  constraint coincident L19.end L20.start
  constraint coincident L8.start L35.end
extrude "Extrude53" cut sketch "Sketch29" against normal blind 1 contours L0 L35 L36 L37 L39 | L2 L4 L37 L39 | L6 L19 L37 L38 L39 bodies 1
extrude "Extrude54" cut 3 faces at (16.3667, -8.45, 29.1667) (16.3667, -8.45, 31.6872) (12.9333, -8.45, 34.9285) along direction (0, -1, 0) blind 1 on bodies 7 bodies 7
sketch "Sketch30" plane through (0, 0, 0) normal (0, 0, -1) x (-1, 0, 0)
  circle A0 centre (-14.65, -7.3) radius 5.3
  line L0 (-14.65, -7.3) -> (-14.65, 0.0002)
  constraint coincident A0.centre L0.start
  constraint vertical L0
sketch "Sketch31" plane through (0, 0, 0) normal (0, 1, 0) x (-1, 0, 0)
  line L0 (-6, 61.5) -> (-28, 61.5)
  line L1 (-28, 61.5) -> (-28, 9)
  line L2 (-28, 9) -> (-26.6505, 9)
  arc A0 (-26.6495, 9) -> (-26.6505, 9) centre (-26.65, 10) ccw
  line L3 (-26.6495, 9) -> (-6, 9)
  line L4 (-6, 9) -> (-6, 59.95)
  arc A1 (-6, 59.95) -> (-6, 59.9505) centre (-7, 59.95) ccw
  line L5 (-6, 59.9505) -> (-6, 61.5)
  circle A2 centre (-26.65, 59.95) radius 1
  circle A3 centre (-9.0124, 10.1568) radius 1
  arc A4 (-8, 59.95) -> (-8, 59.9495) centre (-9, 59.95) ccw
  line L6 (-8, 59.95) -> (-8, 59.9495)
  line L7 (-26.65, 10) -> (-26.65, 59.95)
  constraint coincident A0.centre L7.start
  constraint coincident A2.centre L7.end
hidden bodies 6
